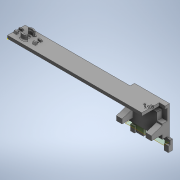
# Autodesk Inventor part: Arm Bottom Left
Saved by Autodesk Inventor 2020.5 (Build 245400000, 400)
## iProperties
Created: 2023-03-21
Part Number: Arm Bottom Left
Material: Generic
Document SubType Name: Modeling
Designer: Wes
Density: 1 g/cm^3
Appearance: Default
Author: Wes
Autodesk Inventor part; units mm, degrees
ref_plane "YZ Plane" through (0, 0, 0) normal (1, 0, 0) x (0, 1, 0)
ref_plane "XZ Plane" through (0, 0, 0) normal (0, 1, 0) x (-1, 0, 0)
ref_plane "XY Plane" through (0, 0, 0) normal (0, 0, 1) x (1, 0, 0)
sketch "Base" plane through (0, 0, 0) normal (0, 0, 1) x (1, 0, 0)
  line L0 (0, 0) -> (-30, 0)
  line L1 (-30, 0) -> (-30, 230)
  line L2 (-30, 230) -> (0, 230)
  line L3 (0, 230) -> (0, 0)
  dimension "d0" = 30
  dimension "d1" = 230
  constraints: 8 end point, 2 parallel, 1 horizontal, 1 perpendicular
  measures "d0" distance of L1.end L2.end
  measures "d1" distance of L0.end L1.end
sketch "Base outline for Extrusion1" plane through (0, 0, 0) normal (0, 0, 1) x (1, 0, 0)
  line L0 (0, 0) -> (0, 230)
  line L1 (-30, 0) -> (0, 0)
  line L2 (-30, 230) -> (-30, 0)
  line L3 (0, 230) -> (-30, 230)
extrude "Extrusion1" add sketch "Base outline for Extrusion1" along normal blind 5
sketch "Axle Screw Countersink" plane through (0, 0, 5) normal (0, 0, 1) x (1, 0, 0)
  line L0 (-15, 0) -> (-15, 20) construction
  circle A0 centre (-15, 20) radius 3.15
  dimension "d4" = 20
  dimension "d58" = 6.3
  constraints: 2 end point, 1 centre point, 1 coincident, 1 vertical
  measures "d4" distance of L0.start L0.end
  measures "d58" diameter of A0
sketch "Axle Screw Countersink outline for Extrusion2" plane through (0, 0, 5) normal (0, 0, 1) x (1, 0, 0)
  circle A0 centre (-15, 20) radius 3.15
extrude "Extrusion2" cut sketch "Axle Screw Countersink outline for Extrusion2" against normal blind 1.2
sketch "Motor Arm Center Fitting" plane through (0, 0, 5) normal (0, 0, 1) x (1, 0, 0)
  line L0 (-19.392963, 15.95) -> (-19.392963, 24.05) construction
  arc A0 (-19.392963, 24.05) -> (-19.392963, 15.95) centre (-15, 20) ccw
  line L1 (-19.392963, 15.95) -> (-21.231023, 14.255439)
  line L2 (-19.392963, 24.05) -> (-21.231023, 25.744561)
  line L3 (-15, 8.350441) -> (-15, 30.698869) construction
  arc A1 (-21.231023, 25.744561) -> (-21.231023, 14.255439) centre (-15, 20) ccw
  line L4 (-10.607037, 15.95) -> (-10.607037, 24.05) construction
  line L5 (-10.607037, 15.95) -> (-19.392963, 15.95) construction
  arc A2 (-10.607037, 15.95) -> (-10.607037, 24.05) centre (-15, 20) ccw
  line L6 (-10.607037, 15.95) -> (-8.768977, 14.255439)
  line L7 (-10.607037, 24.05) -> (-8.768977, 25.744561)
  arc A3 (-8.768977, 14.255439) -> (-8.768977, 25.744561) centre (-15, 20) ccw
  circle A4 centre (-15, 20) radius 5.975 construction
  point P0 (0, 0)
  point P1 (-15, 20)
  dimension "d18" = 11.95
  dimension "d19" = 8.1
  dimension "d20" = 8.1
  dimension "d21" = 2.5
  dimension "d22" = 2.5
  constraints: 16 end point, 12 point on circle, 5 centre point, 2 line through centre, 2 symmetric about line, 2 vertical, 1 concentric, 1 perpendicular, 2 other
  measures "d18" diameter of A4
  measures "d19" distance of L5.start L4.end
  measures "d20" distance of L5.end L0.end
  measures "d21" distance of L5.end L1.end
  measures "d22" distance of L0.end L2.end
sketch "Motor Arm Center Fitting outline for Extrusion3" plane through (0, 0, 5) normal (0, 0, 1) x (1, 0, 0)
  arc A0 (-10.607037, 24.05) -> (-10.607037, 15.95) centre (-15, 20) cw
  line L0 (-8.768977, 25.744561) -> (-10.607037, 24.05)
  arc A1 (-8.768977, 14.255439) -> (-8.768977, 25.744561) centre (-15, 20) ccw
  line L1 (-10.607037, 15.95) -> (-8.768977, 14.255439)
  arc A2 (-21.231023, 25.744561) -> (-21.231023, 14.255439) centre (-15, 20) ccw
  line L2 (-19.392963, 24.05) -> (-21.231023, 25.744561)
  arc A3 (-19.392963, 15.95) -> (-19.392963, 24.05) centre (-15, 20) cw
  line L3 (-21.231023, 14.255439) -> (-19.392963, 15.95)
extrude "Extrusion3" add sketch "Motor Arm Center Fitting outline for Extrusion3" along normal blind 5
sketch "Motor Rotation Support" plane through (0, 0, 10) normal (0, 0, 1) x (1, 0, 0)
  line L0 (-20.975, 20) -> (-21.775, 20) construction
  circle A0 centre (-15, 20) radius 6.775 construction
  arc A1 (-19.981142, 24.592259) -> (-19.981142, 15.407741) centre (-15, 20) ccw
  line L1 (-21.775, 20) -> (-23.775, 20) construction
  circle A2 centre (-15, 20) radius 8.775 construction
  arc A3 (-21.45159, 25.947908) -> (-21.45159, 14.052092) centre (-15, 20) ccw
  line L2 (-21.45159, 14.052092) -> (-19.981142, 15.407741)
  line L3 (-19.981142, 24.592259) -> (-21.45159, 25.947908)
  line L4 (-15, 8.529475) -> (-15, 32.047921) construction
  line L5 (-8.54841, 14.052092) -> (-10.018858, 15.407741)
  arc A4 (-8.54841, 14.052092) -> (-8.54841, 25.947908) centre (-15, 20) ccw
  arc A5 (-10.018858, 15.407741) -> (-10.018858, 24.592259) centre (-15, 20) ccw
  line L6 (-10.018858, 24.592259) -> (-8.54841, 25.947908)
  point P0 (0, 0)
  point P1 (-21.231023, 14.255439)
  point P2 (-21.231023, 25.744561)
  dimension "d25" = 0.8
  dimension "d26" = 2
  constraints: 16 point on circle, 14 end point, 6 centre point, 4 symmetric about line, 2 coincident, 2 horizontal, 1 concentric, 1 vertical, 2 other
  measures "d25" distance of L0.start L0.end
  measures "d26" distance of L0.end L1.end
sketch "Motor Rotation Support outline for Extrusion4" plane through (0, 0, 10) normal (0, 0, 1) x (1, 0, 0)
  arc A0 (-8.54841, 14.052092) -> (-8.54841, 25.947908) centre (-15, 20) ccw
  line L0 (-10.018858, 15.407741) -> (-8.54841, 14.052092)
  arc A1 (-10.018858, 24.592259) -> (-10.018858, 15.407741) centre (-15, 20) cw
  line L1 (-8.54841, 25.947908) -> (-10.018858, 24.592259)
  arc A2 (-21.45159, 25.947908) -> (-21.45159, 14.052092) centre (-15, 20) ccw
  line L2 (-19.981142, 24.592259) -> (-21.45159, 25.947908)
  arc A3 (-19.981142, 15.407741) -> (-19.981142, 24.592259) centre (-15, 20) cw
  line L3 (-21.45159, 14.052092) -> (-19.981142, 15.407741)
extrude "Extrusion4" add sketch "Motor Rotation Support outline for Extrusion4" along normal blind 3.35
sketch "Motor Arm Screw Holes" plane through (0, 0, 5) normal (0, 0, 1) x (1, 0, 0)
  line L0 (-15, 20) -> (-15, 37.1) construction
  line L1 (-15, 20) -> (-15, 2.9) construction
  line L2 (-15, 20) -> (-15, 4.2) construction
  line L3 (-15, 20) -> (-15, 35.8) construction
  line L4 (-15, 4.2) -> (-15, 2.9) construction
  line L5 (-15, 35.8) -> (-15, 37.1) construction
  circle A0 centre (-15, 36.45) radius 1.175
  circle A1 centre (-15, 3.55) radius 1.175
  point P0 (0, 0)
  dimension "d59" = 34.2
  dimension "d60" = 31.6
  dimension "d61" = 2.35
  dimension "d62" = 2.35
  constraints: 12 end point, 3 vertical, 2 centre point, 2 midpoint, 2 point on line, 1 coincident, 1 collinear
  measures "d59" distance of L0.end L1.end
  measures "d60" distance of L3.end L2.end
  measures "d61" diameter of A0
  measures "d62" diameter of A1
sketch "Motor Arm Screw Holes outline for Extrusion5" plane through (0, 0, 5) normal (0, 0, 1) x (1, 0, 0)
  circle A0 centre (-15, 36.45) radius 1.175
  circle A1 centre (-15, 3.55) radius 1.175
extrude "Extrusion5" cut sketch "Motor Arm Screw Holes outline for Extrusion5" against normal through all
sketch "Motor Arm Support" plane through (0, 0, 5) normal (0, 0, 1) x (1, 0, 0)
  line L0 (-15, 2.375) -> (-15, 6.875) construction
  line L1 (-15, 6.875) -> (-11.875, 6.875) construction
  line L2 (-15, 6.875) -> (-18.125, 6.875) construction
  line L3 (-21.064431, 20.215447) -> (-9.114431, 20.215447) construction
  line L4 (-15, 3.55) -> (-12.2, 3.55) construction
  line L5 (-15, 3.55) -> (-12.2, 3.55) construction
  line L6 (-15, 3.55) -> (-17.8, 3.55) construction
  line L7 (-15, 3.55) -> (-12.2, 3.55) construction
  line L8 (-18.125, 6.875) -> (-17.8, 3.55)
  line L9 (-17.8, 3.55) -> (-19.790514, 3.355438)
  line L10 (-19.790514, 3.355438) -> (-20.115514, 6.680438)
  line L11 (-20.115514, 6.680438) -> (-18.125, 6.875)
  line L12 (-11.875, 6.875) -> (-12.2, 3.55)
  line L13 (-12.2, 3.55) -> (-10.209486, 3.355438)
  line L14 (-9.884486, 6.680438) -> (-11.875, 6.875)
  line L15 (-10.209486, 3.355438) -> (-9.884486, 6.680438)
  line L16 (-17.8, 3.55) -> (-17.605438, 1.559486)
  line L17 (-17.605438, 1.559486) -> (-19.595952, 1.364925)
  line L18 (-19.595952, 1.364925) -> (-19.790514, 3.355438)
  line L19 (-12.2, 3.55) -> (-12.394562, 1.559486)
  line L20 (-12.394562, 1.559486) -> (-10.404048, 1.364925)
  line L21 (-10.404048, 1.364925) -> (-10.209486, 3.355438)
  line L22 (-17.8, 36.880894) -> (-19.790514, 37.075456)
  line L23 (-17.8, 36.880894) -> (-17.605438, 38.871408)
  line L24 (-17.605438, 38.871408) -> (-19.595952, 39.06597)
  line L25 (-19.595952, 39.06597) -> (-19.790514, 37.075456)
  line L26 (-18.125, 33.555894) -> (-17.8, 36.880894)
  line L27 (-19.790514, 37.075456) -> (-20.115514, 33.750456)
  line L28 (-20.115514, 33.750456) -> (-18.125, 33.555894)
  line L29 (-11.875, 33.555894) -> (-12.2, 36.880894)
  line L30 (-12.394562, 38.871408) -> (-10.404048, 39.06597)
  line L31 (-12.2, 36.880894) -> (-10.209486, 37.075456)
  line L32 (-10.404048, 39.06597) -> (-10.209486, 37.075456)
  line L33 (-10.209486, 37.075456) -> (-9.884486, 33.750456)
  line L34 (-9.884486, 33.750456) -> (-11.875, 33.555894)
  line L35 (-12.2, 36.880894) -> (-12.394562, 38.871408)
  point P0 (0, 0)
  dimension "d63" = 4.5
  dimension "d64" = 6.25
  dimension "d65" = 5.6
  dimension "d66" = 2
  dimension "d67" = 2
  constraints: 72 end point, 18 symmetric about line, 7 horizontal, 5 perpendicular, 2 collinear, 1 vertical
  measures "d63" distance of L0.start L1.start
  measures "d64" distance of L2.end L1.end
  measures "d65" distance of L8.end L4.end
  measures "d66" distance of L8.end L10.start
  measures "d67" distance of L8.end L17.start
sketch "Motor Arm Support outline for Extrusion6" plane through (0, 0, 5) normal (0, 0, 1) x (1, 0, 0)
  line L0 (-11.875, 6.875) -> (-12.394562, 1.559486)
  line L1 (-12.394562, 1.559486) -> (-10.404048, 1.364925)
  line L2 (-10.404048, 1.364925) -> (-9.884486, 6.680438)
  line L3 (-9.884486, 6.680438) -> (-11.875, 6.875)
  line L4 (-20.115514, 6.680438) -> (-19.595952, 1.364925)
  line L5 (-19.595952, 1.364925) -> (-17.605438, 1.559486)
  line L6 (-17.605438, 1.559486) -> (-18.125, 6.875)
  line L7 (-18.125, 6.875) -> (-20.115514, 6.680438)
  line L8 (-9.884486, 33.750456) -> (-10.404048, 39.06597)
  line L9 (-10.404048, 39.06597) -> (-12.394562, 38.871408)
  line L10 (-12.394562, 38.871408) -> (-11.875, 33.555894)
  line L11 (-11.875, 33.555894) -> (-9.884486, 33.750456)
  line L12 (-18.125, 33.555894) -> (-17.605438, 38.871408)
  line L13 (-17.605438, 38.871408) -> (-19.595952, 39.06597)
  line L14 (-19.595952, 39.06597) -> (-20.115514, 33.750456)
  line L15 (-20.115514, 33.750456) -> (-18.125, 33.555894)
extrude "Extrusion6" add sketch "Motor Arm Support outline for Extrusion6" along normal blind 3
draft "FaceDraft1" angle 28 pull direction (0, 0, 1) faces at (-10.23086, 3.136763, 6) (-10.057673, 35.522294, 6) fixed edges at (-10.144267, 4.022682, 8) (-10.144267, 36.408213, 8)
draft "FaceDraft2" angle 28 pull direction (0, 0, 1) faces at (-19.76914, 37.294132, 6) (-19.942327, 4.9086, 6) fixed edges at (-19.855733, 36.408213, 8) (-19.855733, 4.022682, 8)
fillet "Fillet1" radius 2 4 edges at (-23.475, 20, 5) (-6.525, 20, 5) (-8.225, 20, 10) (-21.775, 20, 10)
sketch "Axle Hole" plane through (0, 0, 5) normal (0, 0, 1) x (1, 0, 0)
  line L0 (0, 230) -> (-30, 230) construction
  line L1 (-15, 230) -> (-15, 220) construction
  circle A0 centre (-15, 220) radius 1.5
  point P0 (0, 0)
  dimension "d73" = 10
  dimension "d74" = 3
  constraints: 2 end point, 1 centre point, 1 coincident, 1 midpoint, 1 vertical
  measures "d73" distance of L1.start L1.end
  measures "d74" diameter of A0
sketch "Axle Hole outline for Extrusion7" plane through (0, 0, 5) normal (0, 0, 1) x (1, 0, 0)
  circle A0 centre (-15, 220) radius 1.5
extrude "Extrusion7" cut sketch "Axle Hole outline for Extrusion7" against normal through all
sketch "Motor Backplate Offset" plane through (0, 0, 0) normal (0, 0, -1) x (-1, 0, 0)
  circle A0 centre (15, 220) radius 1.5 construction
  line L0 (15, 220) -> (15, 180) construction
  line L1 (15, 220) -> (15, 240) construction
  line L2 (30, 240) -> (33.5, 240)
  line L3 (33.5, 240) -> (33.5, 180)
  line L4 (33.5, 180) -> (30, 180)
  line L5 (30, 180) -> (30, 240)
  point P0 (0, 0)
  dimension "d77" = 40
  dimension "d78" = 20
  dimension "d83" = 3.5
  dimension "d84" = 60
  constraints: 12 end point, 2 parallel, 2 vertical, 1 horizontal, 1 perpendicular
  measures "d77" distance of L0.start L0.end
  measures "d78" distance of L0.start L1.end
  measures "d83" distance of L3.end L4.end
  measures "d84" distance of L0.end L1.end
sketch "Motor Backplate Offset outline for Extrusion8" plane through (0, 0, 0) normal (0, 0, -1) x (-1, 0, 0)
  line L0 (30, 240) -> (30, 180)
  line L1 (33.5, 240) -> (30, 240)
  line L2 (33.5, 180) -> (33.5, 240)
  line L3 (30, 180) -> (33.5, 180)
extrude "Extrusion8" add sketch "Motor Backplate Offset outline for Extrusion8" against normal up to surface (5 mm away)
sketch "Motor Backplate" plane through (0, 0, 0) normal (0, 0, -1) x (-1, 0, 0)
  line L0 (33.5, 180) -> (33.5, 240) projected
  line L1 (33.5, 240) -> (37.5, 240)
  line L2 (37.5, 240) -> (37.5, 180)
  line L3 (37.5, 180) -> (33.5, 180)
  line L4 (33.5, 180) -> (33.5, 240)
  point P0 (0, 0)
  dimension "d85" = 4
  constraints: 8 end point, 2 parallel, 1 horizontal, 1 perpendicular
  measures "d85" distance of L2.end L3.end
sketch "Motor Backplate outline for Extrusion9" plane through (0, 0, 0) normal (0, 0, -1) x (-1, 0, 0)
  line L0 (33.5, 180) -> (37.5, 180)
  line L1 (33.5, 240) -> (33.5, 180)
  line L2 (37.5, 240) -> (33.5, 240)
  line L3 (37.5, 180) -> (37.5, 240)
extrude "Extrusion9" add sketch "Motor Backplate outline for Extrusion9" along normal blind 62 and the other way blind 5
sketch "Reference" plane through (0, 0, 0) normal (0, 0, -1) x (-1, 0, 0)
  circle A0 centre (15, 220) radius 1.5 construction
  line L0 (15, 220) -> (24.935, 220) construction
  point P0 (0, 0)
  dimension "d98" = 9.935
  constraints: 2 end point, 1 horizontal
  measures "d98" distance of L0.start L0.end
sketch "Motor Riser" plane through (-33.5, 180, 0) normal (1, 0, 0) x (0, 0, -1)
  line L0 (0, 30) -> (6, 30) construction
  line L1 (6, 30) -> (42, 30) construction
  line L2 (-5, 60) -> (62, 60) projected
  line L3 (42, 60) -> (19, 60)
  line L4 (19, 60) -> (19, 0)
  line L5 (19, 0) -> (42, 0)
  line L6 (42, 0) -> (42, 60)
  line L7 (6, 30) -> (6, 51)
  line L8 (6, 30) -> (6, 9)
  line L9 (6, 51) -> (19, 51)
  line L10 (6, 9) -> (19, 9)
  point P0 (0, -180)
  dimension "d90" = 6
  dimension "d92" = 36
  dimension "d93" = 23
  dimension "d94" = 60
  dimension "d97" = 42
  constraints: 20 end point, 3 horizontal, 3 perpendicular, 3 point on line, 2 parallel, 2 vertical
  measures "d90" distance of L0.start L0.end
  measures "d92" distance of L0.end L1.end
  measures "d93" distance of L5.end L4.end
  measures "d94" distance of L4.end L3.end
  measures "d97" distance of L8.end L7.end
sketch "Motor Riser outline for Extrusion10" plane through (-33.5, 180, 0) normal (1, 0, 0) x (0, 0, -1)
  line L0 (6, 30) -> (6, 9)
  line L1 (6, 51) -> (6, 30)
  line L2 (19, 51) -> (6, 51)
  line L3 (19, 60) -> (19, 51)
  line L4 (42, 60) -> (19, 60)
  line L5 (42, 0) -> (42, 60)
  line L6 (19, 0) -> (42, 0)
  line L7 (19, 9) -> (19, 0)
  line L8 (6, 9) -> (19, 9)
extrude "Extrusion10" add sketch "Motor Riser outline for Extrusion10" along normal up to surface (8.565 mm away)
sketch "Motor Attachment Towers" plane through (-24.935, 180, -42) normal (1, 0, 0) x (0, 0, -1)
  line L0 (0, 60) -> (0, 0) construction
  line L1 (0, 30) -> (-7, 30) construction
  line L2 (-7, 30) -> (-7, 9.8) construction
  line L3 (-7, 30) -> (-7, 50.2) construction
  line L4 (-7, 9.8) -> (-14.5, 9.8)
  line L5 (-14.5, 9.8) -> (-14.5, 0)
  line L6 (-14.5, 0) -> (-7, 0)
  line L7 (-7, 0) -> (-7, 9.8)
  line L8 (-47, 60) -> (20, 60) projected
  line L9 (-7, 50.2) -> (-14.5, 50.2)
  line L10 (-14.5, 50.2) -> (-14.5, 60)
  line L11 (-14.5, 60) -> (-7, 60)
  line L12 (-7, 60) -> (-7, 50.2)
  point P0 (-42, -180)
  point P1 (-7, 60)
  dimension "d101" = 7
  dimension "d102" = 20.2
  dimension "d104" = 40.4
  dimension "d105" = 7.5
  dimension "d106" = 9.8
  constraints: 22 end point, 4 parallel, 3 horizontal, 2 perpendicular, 2 vertical, 1 midpoint, 1 point on line
  measures "d101" distance of L1.start L1.end
  measures "d102" distance of L1.end L2.end
  measures "d104" distance of L3.end L2.end
  measures "d105" distance of L6.end L5.end
  measures "d106" distance of L5.end L4.end
sketch "Motor Attachment Towers outline for Extrusion11" plane through (-24.935, 180, -42) normal (1, 0, 0) x (0, 0, -1)
  line L0 (-14.5, 50.2) -> (-7, 50.2)
  line L1 (-14.5, 60) -> (-14.5, 50.2)
  line L2 (-7, 60) -> (-14.5, 60)
  line L3 (-7, 50.2) -> (-7, 60)
  line L4 (-7, 9.8) -> (-14.5, 9.8)
  line L5 (-7, 0) -> (-7, 9.8)
  line L6 (-14.5, 0) -> (-7, 0)
  line L7 (-14.5, 9.8) -> (-14.5, 0)
extrude "Extrusion11" add sketch "Motor Attachment Towers outline for Extrusion11" along normal blind 18.5
sketch "Motor Screw Holes" plane through (-24.935, 180, -35) normal (0, 0, -1) x (-1, 0, 0)
  circle A0 centre (-9.935, 40) radius 1.5 construction
  line L0 (-9.935, 40) -> (-9.935, 54.55) construction
  line L1 (-9.935, 40) -> (-9.935, 5.7) construction
  line L2 (-9.935, 5.7) -> (-14.845, 5.7) construction
  line L3 (-9.935, 5.7) -> (-5.025, 5.7) construction
  circle A1 centre (-14.845, 5.7) radius 1.275
  circle A2 centre (-5.025, 5.7) radius 1.275
  line L4 (0, 60) -> (0, 0) construction
  line L5 (0, 30) -> (-23.117922, 30) construction
  circle A3 centre (-14.845, 54.3) radius 1.275
  circle A4 centre (-5.025, 54.3) radius 1.275
  point P0 (-24.935, -180)
  dimension "d109" = 14.55
  dimension "d110" = 34.3
  dimension "d111" = 4.91
  dimension "d113" = 9.82
  dimension "d114" = 2.55
  dimension "d115" = 2.55
  constraints: 10 end point, 4 centre point, 3 horizontal, 2 coincident, 2 symmetric about line, 2 vertical, 1 midpoint, 2 other
  measures "d109" distance of L0.start L0.end
  measures "d110" distance of L0.start L1.end
  measures "d111" distance of L1.end L2.end
  measures "d113" distance of L3.end L2.end
  measures "d114" diameter of A1
  measures "d115" diameter of A2
sketch "Motor Screw Holes outline for Extrusion12" plane through (-24.935, 180, -35) normal (0, 0, -1) x (-1, 0, 0)
  circle A0 centre (-14.845, 5.7) radius 1.275
  circle A1 centre (-14.845, 54.3) radius 1.275
  circle A2 centre (-5.025, 5.7) radius 1.275
  circle A3 centre (-5.025, 54.3) radius 1.275
extrude "Extrusion12" cut sketch "Motor Screw Holes outline for Extrusion12" against normal blind 4
draft "FaceDraft3" angle 18 pull direction (1, 0, 0) faces at (-18.768333, 236.733333, -27.5) (-18.768333, 186.533333, -27.5) fixed edges at (-6.435, 235.1, -27.5) (-6.435, 184.9, -27.5)
ref_plane "Arm Clearance Offset Plane" through (-33.5, 180, -49) normal (0, 0, -1) x (-1, 0, 0)
sketch "Arm Clearance Cut" plane through (-33.5, 180, -49) normal (0, 0, -1) x (-1, 0, 0)
  circle A0 centre (-18.5, 40) radius 1.5 construction
  line L0 (-18.5, 40) -> (-0.823054, 30.644489) construction
  line L1 (-14.673289, 21.324047) -> (-88.916461, 60.617195)
  line L2 (-92.245035, 71.430177) -> (-85.696177, 83.804039)
  line L3 (-74.883194, 87.132613) -> (-0.640022, 47.839466)
  line L4 (2.688552, 37.026483) -> (-3.860306, 24.652621)
  arc A1 (-92.245035, 71.430177) -> (-88.916461, 60.617195) centre (-85.174256, 67.687973) ccw
  arc A2 (-74.883194, 87.132613) -> (-85.696177, 83.804039) centre (-78.625399, 80.061835) ccw
  arc A3 (-14.673289, 21.324047) -> (-3.860306, 24.652621) centre (-10.931084, 28.394826) ccw
  arc A4 (2.688552, 37.026483) -> (-0.640022, 47.839466) centre (-4.382227, 40.768688) ccw
  line L5 (-8.565, 9) -> (-8.565, 51) construction
  line L6 (-8.565, 19.239602) -> (4, 19.239602) construction
  line L7 (4, 60) -> (4, 0) construction
  line L8 (0, 51) -> (0, 60) construction
  line L9 (0, 60) -> (0, 56) construction
  line L10 (0, 9) -> (0, 51)
  line L11 (0, 19.239602) -> (4, 19.239602)
  line L12 (4, 19.239602) -> (4, 56)
  line L13 (4, 56) -> (0, 56)
  line L14 (0, 56) -> (0, 19.239602)
  point P0 (-33.5, -180)
  point P1 (-81.953972, 90.874818)
  point P2 (-95.987239, 64.359399)
  point P3 (6.430756, 44.097262)
  dimension "d119" = 20
  dimension "d120" = 100
  dimension "d121" = 30
  dimension "d122" = 8
  dimension "d124" = 4
  constraints: 22 end point, 12 point on line, 8 point on circle, 8 tangent, 4 centre point, 4 parallel, 3 equal radius, 2 horizontal, 2 perpendicular
  measures "d119" distance of A0.centre L0.end
  measures "d120" distance of point (-81.954, 90.875) point (6.431, 44.097)
  measures "d121" distance of point (-95.987, 64.359) point (-81.954, 90.875)
  measures "d122" radius of A1
  measures "d124" distance of L8.end L9.end
sketch "Arm Clearance Cut outline for Extrusion13" plane through (-33.5, 180, -49) normal (0, 0, -1) x (-1, 0, 0)
  line L0 (4, 56) -> (0, 56)
  line L1 (4, 19.239602) -> (4, 56)
  line L2 (0, 19.239602) -> (4, 19.239602)
  line L3 (0, 51) -> (0, 19.239602)
  line L4 (0, 56) -> (0, 51)
extrude "Extrusion13" cut sketch "Arm Clearance Cut outline for Extrusion13" along normal up to surface (13 mm away)
sketch "Connector Support" plane through (-33.5, 180, -49) normal (0, 0, -1) x (-1, 0, 0)
  line L0 (4, 60) -> (0, 60) projected
  line L1 (4, 60) -> (0, 60)
  line L2 (0, 60) -> (0, 65)
  line L3 (0, 65) -> (4, 65)
  line L4 (4, 65) -> (4, 60)
  point P0 (-33.5, -180)
  dimension "d127" = 5
  constraints: 8 end point, 2 parallel, 1 horizontal, 1 perpendicular
  measures "d127" distance of L1.end L2.end
sketch "Connector Support outline for Extrusion14" plane through (-33.5, 180, -49) normal (0, 0, -1) x (-1, 0, 0)
  line L0 (4, 60) -> (4, 65)
  line L1 (0, 60) -> (4, 60)
  line L2 (0, 65) -> (0, 60)
  line L3 (4, 65) -> (0, 65)
extrude "Extrusion14" add sketch "Connector Support outline for Extrusion14" along normal blind 13 and the other way blind 4
sketch "Connector Screw Support" plane through (0, 0, -62) normal (0, 0, -1) x (-1, 0, 0)
  line L0 (33.5, 180) -> (33.5, 189) projected
  line L1 (33.5, 180) -> (30.5, 180)
  line L2 (30.5, 180) -> (30.5, 187)
  line L3 (30.5, 187) -> (33.5, 187)
  line L4 (33.5, 187) -> (33.5, 180)
  line L5 (33.5, 245) -> (33.5, 236) projected
  line L6 (33.5, 245) -> (30.5, 245)
  line L7 (30.5, 245) -> (30.5, 238)
  line L8 (30.5, 238) -> (33.5, 238)
  line L9 (33.5, 238) -> (33.5, 245)
  point P0 (0, 0)
  dimension "d132" = 3
  dimension "d133" = 7
  dimension "d134" = 3
  dimension "d135" = 7
  constraints: 16 end point, 4 parallel, 2 horizontal, 2 perpendicular
  measures "d132" distance of L2.end L3.end
  measures "d133" distance of L1.end L2.end
  measures "d134" distance of L8.end L7.end
  measures "d135" distance of L7.end L6.end
sketch "Connector Screw Support outline for Extrusion15" plane through (0, 0, -62) normal (0, 0, -1) x (-1, 0, 0)
  line L0 (30.5, 245) -> (30.5, 238)
  line L1 (33.5, 245) -> (30.5, 245)
  line L2 (33.5, 238) -> (33.5, 245)
  line L3 (30.5, 238) -> (33.5, 238)
  line L4 (30.5, 187) -> (30.5, 180)
  line L5 (33.5, 187) -> (30.5, 187)
  line L6 (33.5, 180) -> (33.5, 187)
  line L7 (30.5, 180) -> (33.5, 180)
extrude "Extrusion15" add sketch "Connector Screw Support outline for Extrusion15" against normal blind 10
sketch "Connector Screw Holes" plane through (0, 0, -62) normal (0, 0, -1) x (-1, 0, 0)
  line L0 (30.5, 180) -> (30.5, 187) projected
  line L1 (30.5, 238) -> (30.5, 245) projected
  circle A0 centre (34, 183.5) radius 1.275
  circle A1 centre (34, 241.5) radius 1.275
  point P0 (0, 0)
  point P1 (30.5, 183.5)
  point P2 (30.5, 241.5)
  dimension "d138" = 2.55
  dimension "d139" = 2.55
  constraints: 2 centre point, 2 midpoint
  measures "d138" diameter of A0
  measures "d139" diameter of A1
sketch "Connector Screw Holes outline for Extrusion16" plane through (0, 0, -62) normal (0, 0, -1) x (-1, 0, 0)
  circle A0 centre (34, 183.5) radius 1.275
  circle A1 centre (34, 241.5) radius 1.275
extrude "Extrusion16" cut sketch "Connector Screw Holes outline for Extrusion16" against normal blind 10
body "Solid1"
